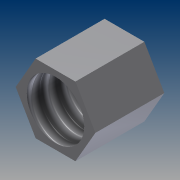
# Autodesk Inventor part: standoffiPart-01
Saved by Autodesk Inventor 2011 SP1 (Build 150282100, 282)
## iProperties
Created: 2011-07-21
Part Number: standoffiPart-01
Document SubType Name: Modeling
Designer: Nathan
Density: 1 g/cm^3
Author: Nathan
Autodesk Inventor part; units mm, degrees
ref_plane "YZ Plane" through (0, 0, 0) normal (1, 0, 0) x (0, 1, 0)
ref_plane "XZ Plane" through (0, 0, 0) normal (0, 1, 0) x (-1, 0, 0)
ref_plane "XY Plane" through (0, 0, 0) normal (0, 0, 1) x (1, 0, 0)
sketch "Sketch1" plane through (0, 0, 0) normal (0, 0, 1) x (1, 0, 0)
  line L0 (1.8331, 0) -> (0.9165, -1.5875)
  line L1 (0.9165, -1.5875) -> (-0.9165, -1.5875)
  line L2 (-0.9165, -1.5875) -> (-1.8331, 0)
  line L3 (-1.8331, 0) -> (-0.9165, 1.5875)
  line L4 (-0.9165, 1.5875) -> (0.9165, 1.5875)
  line L5 (0.9165, 1.5875) -> (1.8331, 0)
  point P0 (0, 0)
  point P1 (0, 0)
  dimension "Diameter" = 3.175
  constraints: 12 end point, 1 coincident, 13 other
  measures "Diameter" distance between parallel lines of L4 L1
extrude "Extrusion1" add sketch "Sketch1" along normal blind 3.175
sketch "Sketch2" plane through (0, 0, 3.175) normal (0, 0, 1) x (1, 0, 0)
  point P0 (0, 0)
  point P1 (0, 0)
  constraints: 1 coincident
hole "Hole1" at (0, 0, 3.175) direction (0, 0, -1) diameter 2.6416 end through all thread size "6-32 UNC" class "2B" standard "ANSI Unified Screw Threads"
body "Solid1"
